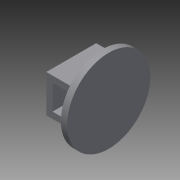
# Autodesk Inventor part: foot_holder
Saved by Autodesk Inventor 2015 SP1 (Build 190203100, 203)
## iProperties
Created: 2015-07-17
Part Number: foot_holder
Material: Generic
Document SubType Name: Modeling
Designer: Alexandre Cherpillod
Density: 1 g/cm^3
Appearance: Default
Author: Alexandre Cherpillod
Autodesk Inventor part; units mm, degrees
ref_plane "YZ Plane" through (0, 0, 0) normal (1, 0, 0) x (0, 1, 0)
ref_plane "XZ Plane" through (0, 0, 0) normal (0, 1, 0) x (-1, 0, 0)
ref_plane "XY Plane" through (0, 0, 0) normal (0, 0, 1) x (1, 0, 0)
sketch "Sketch1" plane through (0, 0, 0) normal (1, 0, 0) x (0, 1, 0)
  circle A0 centre (0, 0) radius 10
  dimension "d0" = 20
  constraints: 1 centre point, 1 coincident
  measures "d0" diameter of A0
extrude "Extrusion1" add sketch "Sketch1" along normal blind 1.5
sketch "Sketch2" plane through (0, 0, 0) normal (-1, 0, 0) x (0, 0, 1)
  line L0 (4.5, -6) -> (-4.5, -6)
  line L1 (-4.5, -6) -> (-4.5, 6)
  line L2 (-4.5, 6) -> (4.5, 6)
  line L3 (4.5, 6) -> (4.5, -6)
  line L4 (4.5, -6) -> (-4.5, 6) construction
  line L5 (-4.5, -6) -> (4.5, 6) construction
  point P0 (0, 0)
  dimension "d3" = 9
  dimension "d4" = 12
  constraints: 12 end point, 2 midpoint, 2 parallel, 1 horizontal, 1 perpendicular
  measures "d3" distance of L1.end L2.end
  measures "d4" distance of L0.end L1.end
extrude "Extrusion2" add sketch "Sketch2" along normal blind 7.5
sketch "Sketch3" plane through (0, 6, 4.5) normal (0, 1, 0) x (1, 0, 0)
  line L0 (-6, 1.5) -> (0, 1.5)
  line L1 (0, 1.5) -> (0, 7.5)
  line L2 (0, 7.5) -> (-6, 7.5)
  line L3 (-6, 7.5) -> (-6, 1.5)
  line L4 (-6, 1.5) -> (0, 7.5) construction
  line L5 (0, 1.5) -> (-6, 7.5) construction
  line L6 (0, 4.5) -> (-7.5, 4.5) construction
  line L7 (-7.5, 9) -> (-7.5, 0) construction
  line L8 (0, 14.5) -> (0, -5.5) construction
  point P0 (-3, 4.5)
  point P1 (-3, 4.5)
  dimension "d7" = 0
  dimension "d8" = 6
  dimension "d9" = 6
  constraints: 14 end point, 4 midpoint, 2 parallel, 1 horizontal, 1 perpendicular, 1 point on line
  measures "d7" distance between parallel lines of L1 L8
  measures "d8" distance of L1.end L2.end
  measures "d9" distance of L2.end L0.start
extrude "Extrusion3" cut sketch "Sketch3" against normal through all
fillet "Fillet1" radius 2 2 edges at (0, 0, -4.5) (0, 0, 4.5)
body "Solid1"
